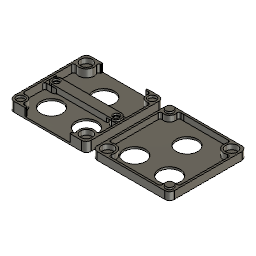
シノン_髪飾り_mk1_v8 (Autodesk Fusion 360 design; units mm, degrees)
Autodesk Fusion 360 part; units mm, degrees
note: some values were not read from the file. Set by a fixed rule: which face or edge a step refers to.
sketch "スケッチ1" plane through (0, 0, 0) normal (0, 0, 1) x (1, 0, 0)
  line L0 (20, 20) -> (-20, 20)
  line L1 (-20, 20) -> (-20, -20)
  line L2 (-20, -20) -> (20, -20)
  line L3 (20, -20) -> (20, 20)
  line L4 (20, 20) -> (-20, -20) construction
  line L5 (-20, 20) -> (20, -20) construction
  circle A0 centre (0, 9) radius 5.5
  circle A1 centre (-9, -9) radius 5.5
  circle A2 centre (9, -9) radius 5.5
  line L6 (0, 0) -> (0, 9) construction
  dimension "d1" = 40
  dimension "d2" = 40
  dimension "d3" = 11
  dimension "d4" = 11
  dimension "d5" = 11
  dimension "d7" = 11
  dimension "d8" = 11
  dimension "d9" = 11
  constraint horizontal L0
  constraint perpendicular L0 L1
  constraint parallel L0 L2
  constraint parallel L1 L3
  constraint coincident L4 L6.start
  constraint coincident L5 L6.start
  constraint coincident L6.start origin
  constraint coincident L4 A1.centre
  constraint coincident L5 A2.centre
  constraint coincident A0.centre L6.end
  constraint vertical L6
  measures "d1" distance of L1.end L2.end
  measures "d2" distance of L0.end L1.end
  measures "d3" diameter of A1
  measures "d4" diameter of A2
  measures "d5" diameter of A0
  measures "d7" distance of L1 A1.centre
  measures "d8" distance of L3 A2.centre
  measures "d9" distance of L0 A0.centre
extrude "押し出し1" add sketch "スケッチ1" along normal blind 4 makes body 1
sketch "スケッチ2" plane through (0, 0, 4) normal (0, 0, 1) x (-1, 0, 0)
  circle A0 centre (0, -9) radius 5.5
  circle A1 centre (9, 9) radius 5.5
  circle A2 centre (-9, 9) radius 5.5
  line L0 (-20, 20) -> (-20, -20)
  line L1 (-20, -20) -> (20, -20)
  line L2 (20, -20) -> (20, 20)
  line L3 (20, 20) -> (-20, 20)
  line L4 (-19, -19) -> (19, -19)
  line L5 (19, -19) -> (19, 19)
  line L6 (19, 19) -> (-19, 19)
  line L7 (-19, 19) -> (-19, -19)
  line L8 (-19, -19) -> (19, 19) construction
  line L9 (19, -19) -> (-19, 19) construction
  dimension "d12" = 1
  dimension "d13" = 1
  constraint horizontal L4
  constraint perpendicular L4 L5
  constraint parallel L4 L6
  constraint parallel L5 L7
  constraint coincident L8 origin
  constraint coincident L9 origin
  measures "d12" distance of L0 L7
  measures "d13" distance of L1 L4
extrude "押し出し2" cut sketch "スケッチ2" against normal blind 3 contours L4 L5 L6 L7 bodies 1
sketch "スケッチ3" plane through (0, 0, 1) normal (0, 0, 1) x (-1, 0, 0)
  circle A0 centre (-9, 9) radius 5.5
  circle A1 centre (0, -9) radius 5.5
  circle A2 centre (9, 9) radius 5.5
  line L0 (-19, 19) -> (-19, -19)
  line L1 (-19, -19) -> (19, -19)
  line L2 (19, -19) -> (19, 19)
  line L3 (19, 19) -> (-19, 19)
  circle A3 centre (15.5, 0) radius 2.5
  line L4 (19, 0) -> (-19, 0) construction
  circle A4 centre (15.5, 0) radius 1.25
  line L5 (20, -20) -> (20, 20)
  line L6 (0, -19) -> (0, 19)
  line L7 (15.5, -2.5) -> (19, -2.5)
  line L8 (15.5, 2.5) -> (19, 2.5)
  circle A5 centre (-15.5, 0) radius 2.5
  circle A6 centre (-15.5, 0) radius 1.25
  line L9 (-15.5, -2.5) -> (-19, -2.5)
  line L10 (-15.5, 2.5) -> (-19, 2.5)
  dimension "d16" = 5
  dimension "d17" = 2.5
  dimension "d19" = 3.5
  constraint midpoint L2 L4.start
  constraint midpoint L0 L4.end
  constraint coincident A3.centre L4
  constraint concentric A3 A4
  constraint midpoint L1 L6.start
  constraint midpoint L3 L6.end
  constraint coincident A3 L7.start
  constraint coincident L2 L7.end
  constraint perpendicular L2 L7
  constraint coincident A3 L8.start
  constraint coincident L2 L8.end
  constraint perpendicular L2 L8
  constraint tangent A3 L7
  constraint tangent A3 L8
  constraint symmetric A3 L6 A5
  constraint symmetric A4 L6 A6
  constraint symmetric L6 L7.start L9.start
  constraint symmetric L6 L7.end L9.end
  constraint symmetric L6 L8.start L10.start
  constraint symmetric L6 L8.end L10.end
  measures "d16" diameter of A3
  measures "d17" diameter of A4
  measures "d19" distance of L2 A3.centre
extrude "押し出し3" add 1 faces at (-6.3333, 19.6667, 4) along direction (0, 0, 1) blind 1 on bodies 1 bodies 1
extrude "押し出し4" add sketch "スケッチ3" along normal blind 3 contours L2 A3 L7 L8 | L0 A5 L9 L10 | A3 | A5 bodies 1
fillet "フィレット1" radius 2 4 edges at (-19, -19, 3) (19, -19, 3) (19, 19, 3) (-19, 19, 3) on bodies 1
fillet "フィレット2" radius 2.5 4 edges at (20, 20, 2.5) (20, -20, 2.5) (-20, 20, 2.5) (-20, -20, 2.5) on bodies 1
sketch "スケッチ5" plane through (0, 0, 5) normal (0, 0, 1) x (-1, 0, 0)
  line L0 (17, -19) -> (-17, -19)
  arc A0 (-19, -17) -> (-17, -19) centre (-17, -17) ccw
  line L1 (-19, -17) -> (-19, 17)
  arc A1 (-17, 19) -> (-19, 17) centre (-17, 17) ccw
  line L2 (-17, 19) -> (17, 19)
  arc A2 (19, 17) -> (17, 19) centre (17, 17) ccw
  line L3 (19, 17) -> (19, -17)
  arc A3 (17, -19) -> (19, -17) centre (17, -17) ccw
  arc A4 (20, 17.5) -> (17.5, 20) centre (17.5, 17.5) ccw
  line L4 (17.5, 20) -> (-17.5, 20)
  arc A5 (-17.5, 20) -> (-20, 17.5) centre (-17.5, 17.5) ccw
  line L5 (-20, 17.5) -> (-20, -17.5)
  arc A6 (-20, -17.5) -> (-17.5, -20) centre (-17.5, -17.5) ccw
  line L6 (-17.5, -20) -> (17.5, -20)
  arc A7 (17.5, -20) -> (20, -17.5) centre (17.5, -17.5) ccw
  line L7 (20, -17.5) -> (20, 17.5)
extrude "押し出し6" cut 2 faces at (-15.867, 0.0689, 1) (15.2939, 0.4998, 1) along direction (0, 0, -1) blind 1 on bodies 1 bodies 1
fillet "フィレット3" radius 1 4 edges at (19, -2.5, 2.5) (19, 2.5, 2.5) (-19, 2.5, 2.5) (-19, -2.5, 2.5) on bodies 1
sketch "スケッチ6" plane through (0, 0, 1) normal (0, 0, 1) x (-1, 0, 0)
  circle A0 centre (0, -9) radius 5.5
  circle A1 centre (9, 9) radius 5.5
  circle A2 centre (-9, 9) radius 5.5
  arc A3 (18, 2.5) -> (19, 3.5) centre (18, 3.5) ccw
  line L0 (19, 3.5) -> (19, 17)
  arc A4 (19, 17) -> (17, 19) centre (17, 17) ccw
  line L1 (17, 19) -> (-17, 19)
  arc A5 (-17, 19) -> (-19, 17) centre (-17, 17) ccw
  line L2 (-19, 17) -> (-19, 3.5)
  arc A6 (-19, 3.5) -> (-18, 2.5) centre (-18, 3.5) ccw
  line L3 (-18, 2.5) -> (-15.5, 2.5)
  arc A7 (-15.5, -2.5) -> (-15.5, 2.5) centre (-15.5, 0) ccw
  line L4 (-15.5, -2.5) -> (-18, -2.5)
  arc A8 (-18, -2.5) -> (-19, -3.5) centre (-18, -3.5) ccw
  line L5 (-19, -3.5) -> (-19, -17)
  arc A9 (-19, -17) -> (-17, -19) centre (-17, -17) ccw
  line L6 (-17, -19) -> (17, -19)
  arc A10 (17, -19) -> (19, -17) centre (17, -17) ccw
  line L7 (19, -17) -> (19, -3.5)
  arc A11 (19, -3.5) -> (18, -2.5) centre (18, -3.5) ccw
  line L8 (18, -2.5) -> (15.5, -2.5)
  arc A12 (15.5, 2.5) -> (15.5, -2.5) centre (15.5, 0) ccw
  line L9 (15.5, 2.5) -> (18, 2.5)
  circle A13 centre (16, -16) radius 3
  circle A14 centre (16, -16) radius 4
  line L10 (0, 0) -> (0, -19)
  line L11 (15.5, 0) -> (-15.5, 0)
  circle A15 centre (-16, 16) radius 3
  circle A16 centre (-16, 16) radius 4
  line L12 (19, 19) -> (-19, 19)
  line L13 (-19, 19) -> (-19, -19)
  line L14 (13.0505, -0.5) -> (-13.0505, -0.5)
  line L15 (13.0505, 0.5) -> (-13.0505, 0.5)
  dimension "d38" = 6
  dimension "d39" = 8
  dimension "d47" = 6
  dimension "d48" = 8
  dimension "d59" = 0.5
  constraint tangent L6 A13
  constraint tangent L7 A13
  constraint concentric A13 A14
  constraint coincident L10.start origin
  constraint midpoint L6 L10.end
  constraint coincident A12.centre L11.start
  constraint coincident A7.centre L11.end
  constraint tangent A15 L12
  constraint tangent A15 L13
  constraint concentric A15 A16
  constraint coincident A12 L14.start
  constraint coincident A7 L14.end
  constraint parallel L11 L14
  constraint symmetric L11 L14.start L15.start
  constraint symmetric L11 L14.end L15.end
  measures "d38" diameter of A13
  measures "d39" diameter of A14
  measures "d47" diameter of A15
  measures "d48" diameter of A16
  measures "d59" distance of L11 L14
extrude "押し出し9" add sketch "スケッチ6" along normal blind 4 contours L6 L7 A13 A14 | L6 A10 L7 A13 | L1 L2 A15 A16 L12 L13 | L1 A5 L2 A15 L12 L13 bodies 1
fillet "フィレット5" radius 1 4 edges at (-19, 13.3542, 3) (-13.3542, 19, 3) (19, -13.3542, 3) (13.3542, -19, 3) on bodies 1
extrude "押し出し10" add sketch "スケッチ6" along normal blind 1.8 contours A13 | A15 bodies 1
sketch "スケッチ7" plane through (0, 0, 5) normal (0, 0, 1) x (-1, 0, 0)
  line L0 (-19, -17) -> (-19, 11.4174)
  line L1 (19, 17) -> (19, -11.4174)
  arc A0 (20, 17.5) -> (17.5, 20) centre (17.5, 17.5) ccw
  line L2 (17.5, 20) -> (-17.5, 20)
  arc A1 (-17.5, 20) -> (-20, 17.5) centre (-17.5, 17.5) ccw
  line L3 (-20, 17.5) -> (-20, -17.5)
  arc A2 (-20, -17.5) -> (-17.5, -20) centre (-17.5, -17.5) ccw
  line L4 (-17.5, -20) -> (17.5, -20)
  arc A3 (17.5, -20) -> (20, -17.5) centre (17.5, -17.5) ccw
  line L5 (20, -17.5) -> (20, 17.5)
  line L6 (11.4174, -20) -> (11.4174, -19)
  line L7 (0, 0) -> (0, -20)
  line L8 (11.4174, -19) -> (-17, -19)
  arc A4 (-19, -17) -> (-17, -19) centre (-17, -17) ccw
  line L9 (-11.4174, 19) -> (17, 19)
  arc A5 (19, 17) -> (17, 19) centre (17, 17) ccw
  arc A6 (17.6, -12.3339) -> (19, -11.4174) centre (18, -11.4174) ccw
  arc A7 (17.6, -12.3339) -> (12.3339, -17.6) centre (16, -16) ccw
  arc A8 (11.4174, -19) -> (12.3339, -17.6) centre (11.4174, -18) ccw
  arc A9 (-17.6, 12.3339) -> (-19, 11.4174) centre (-18, 11.4174) ccw
  arc A10 (-17.6, 12.3339) -> (-12.3339, 17.6) centre (-16, 16) ccw
  arc A11 (-11.4174, 19) -> (-12.3339, 17.6) centre (-11.4174, 18) ccw
  circle A12 centre (-16, 16) radius 3
  circle A13 centre (16, -16) radius 3
  line L10 (-11.4174, -20) -> (-11.4174, -19)
  line L11 (0, 0) -> (-20, 0)
  line L12 (11.4174, 20) -> (11.4174, 19)
  line L13 (-11.4174, 20) -> (-11.4174, 19)
  constraint coincident L4 L6.start
  constraint coincident L7.start L11.start
  constraint midpoint L4 L7.end
  constraint coincident L6.end L8.start
  constraint symmetric L6.start L7 L10.start
  constraint symmetric L6.end L7 L10.end
  constraint midpoint L3 L11.end
  constraint symmetric L6.start L11 L12.start
  constraint symmetric L6.end L11 L12.end
  constraint symmetric L10.start L11 L13.start
  constraint symmetric L10.end L11 L9.start
extrude "押し出し11" cut sketch "スケッチ7" against normal blind 4 contours L4 L7 L8 L10 | L4 L6 L7 L8 | L2 L9 L12 L13 bodies 1
fillet "フィレット6" radius 0.3 8 edges at (-11.4174, -20, 3) (-11.4174, -19, 3) (11.4174, -20, 3) (-11.4174, 19, 3) (11.4174, 19, 3) (11.4174, 20, 3) (-11.4174, 20, 3) (11.4174, -19, 3) on bodies 1
extrude "押し出し12" add sketch "スケッチ6" along normal blind 1 contours A7 L10 L11 L14 | A12 L10 L11 L14 | A7 A12 L11 L15 bodies 1
fillet "フィレット7" radius 1 4 edges at (-13.0505, -0.5, 1.5) (-13.0505, 0.5, 1.5) (13.0505, 0.5, 1.5) (13.0505, -0.5, 1.5) on bodies 1
mirror "ミラー1" about plane through (0, 0, 5) normal (0, 0, 1) of bodies 1 makes body 2
extrude "押し出し13" cut 1 faces at (-17.8603, 0, 6) along direction (0, 0, 1) blind 3 on bodies 2 bodies 2
extrude "押し出し14" cut 1 faces at (17.8603, 0, 6) along direction (0, 0, 1) blind 3 on bodies 2 bodies 2
extrude "押し出し15" cut 1 faces at (4.1126, -0.1667, 8) along direction (0, 0, 1) blind 1 on bodies 2 bodies 2
sketch "スケッチ8" plane through (0, 0, 9) normal (0, 0, -1) x (1, 0, 0)
  line L0 (19, -17) -> (19, 11.4174)
  arc A0 (19, 11.4174) -> (17.6, 12.3339) centre (18, 11.4174) ccw
  arc A1 (12.3339, 17.6) -> (17.6, 12.3339) centre (16, 16) ccw
  arc A2 (12.3339, 17.6) -> (11.6482, 18.973) centre (11.4174, 18) ccw
  arc A3 (11.4174, 19.2649) -> (11.6482, 18.973) centre (11.7174, 19.2649) ccw
  line L1 (11.4174, 19.2649) -> (11.4174, 19.7)
  arc A4 (11.7174, 20) -> (11.4174, 19.7) centre (11.7174, 19.7) ccw
  line L2 (11.7174, 20) -> (-11.7174, 20)
  arc A5 (-11.4174, 19.7) -> (-11.7174, 20) centre (-11.7174, 19.7) ccw
  line L3 (-11.4174, 19.7) -> (-11.4174, 19.3)
  arc A6 (-11.7174, 19) -> (-11.4174, 19.3) centre (-11.7174, 19.3) ccw
  line L4 (-11.7174, 19) -> (-17, 19)
  arc A7 (-17, 19) -> (-19, 17) centre (-17, 17) ccw
  line L5 (-19, 17) -> (-19, -11.4174)
  arc A8 (-19, -11.4174) -> (-17.6, -12.3339) centre (-18, -11.4174) ccw
  arc A9 (-12.3339, -17.6) -> (-17.6, -12.3339) centre (-16, -16) ccw
  arc A10 (-12.3339, -17.6) -> (-11.6482, -18.973) centre (-11.4174, -18) ccw
  arc A11 (-11.4174, -19.2649) -> (-11.6482, -18.973) centre (-11.7174, -19.2649) ccw
  line L6 (-11.4174, -19.2649) -> (-11.4174, -19.7)
  arc A12 (-11.7174, -20) -> (-11.4174, -19.7) centre (-11.7174, -19.7) ccw
  line L7 (-11.7174, -20) -> (11.7174, -20)
  arc A13 (11.4174, -19.7) -> (11.7174, -20) centre (11.7174, -19.7) ccw
  line L8 (11.4174, -19.7) -> (11.4174, -19.3)
  arc A14 (11.7174, -19) -> (11.4174, -19.3) centre (11.7174, -19.3) ccw
  line L9 (11.7174, -19) -> (17, -19)
  arc A15 (17, -19) -> (19, -17) centre (17, -17) ccw
  circle A16 centre (15.5, 0) radius 1.25
  circle A17 centre (0, -9) radius 5.5
  circle A18 centre (-15.5, 0) radius 1.25
  circle A19 centre (-9, 9) radius 5.5
  circle A20 centre (9, 9) radius 5.5
  circle A21 centre (-15.5, 0) radius 1.25
  circle A22 centre (15.5, 0) radius 1.25
  line L10 (-11.7174, 19) -> (11.6482, 18.973)
  line L11 (-11.6482, -18.973) -> (11.7174, -19)
  constraint concentric A18 A21
  constraint concentric A16 A22
  constraint coincident A6.start L4.start
  constraint coincident A2.end A3.end
  constraint coincident A10.end A11.end
  constraint coincident A14.start L9.start
extrude "押し出し16" add sketch "スケッチ8" along normal blind 4 contours A11 L6 A12 L7 A13 L8 A14 L11 | A3 L1 A4 L2 A5 L3 A6 L10 bodies 2
fillet "フィレット8" radius 1 1 edges at (11.6482, -18.973, 7) on bodies 2
fillet "フィレット9" radius 1 1 edges at (-11.6482, 18.973, 7) on bodies 2
extrude "押し出し17" add sketch "スケッチ8" against normal blind 1 contours A16 A22 | A18 A21 bodies 2
extrude "押し出し18" cut 1 faces at (3.8023, -19.6578, 5) along direction (0, 0, 1) blind 1 on bodies 2 bodies 2
sketch "スケッチ9" plane through (0, 0, 9) normal (0, 0, -1) x (1, 0, 0)
  arc A0 (-12.3247, -17.5786) -> (-11.407, -18.9733) centre (-11.4059, -17.9733) ccw
  line L0 (-11.407, -18.9733) -> (11.7174, -19)
  line L1 (11.7174, -19) -> (17, -19)
  arc A1 (17, -19) -> (19, -17) centre (17, -17) ccw
  line L2 (19, -17) -> (19, 11.4174)
  arc A2 (19, 11.4174) -> (17.6, 12.3339) centre (18, 11.4174) ccw
  arc A3 (12.3247, 17.5786) -> (17.6, 12.3339) centre (16, 16) ccw
  arc A4 (12.3247, 17.5786) -> (11.407, 18.9733) centre (11.4059, 17.9733) ccw
  line L3 (11.407, 18.9733) -> (-11.7174, 19)
  line L4 (-11.7174, 19) -> (-17, 19)
  arc A5 (-17, 19) -> (-19, 17) centre (-17, 17) ccw
  line L5 (-19, 17) -> (-19, -11.4174)
  arc A6 (-19, -11.4174) -> (-17.6, -12.3339) centre (-18, -11.4174) ccw
  arc A7 (-12.3247, -17.5786) -> (-17.6, -12.3339) centre (-16, -16) ccw
  circle A8 centre (0, -9) radius 5.5
  circle A9 centre (-9, 9) radius 5.5
  circle A10 centre (9, 9) radius 5.5
  line L6 (-19, -5) -> (-17.9, -5)
  line L7 (-17.9, -5) -> (-17.9, 20)
  line L8 (-11.7174, 19) -> (-11.7174, 17.9)
  line L9 (-11.7174, 17.9) -> (-17.9, 17.9)
  line L10 (-12.7174, 17.9) -> (-12.7174, 19)
  dimension "d82" = 1.1
  dimension "d83" = 1.1
  dimension "d88" = 1
  constraint coincident L5 L6.start
  constraint perpendicular L5 L6
  constraint perpendicular L6 L7
  constraint coincident L3.end L4.start
  constraint perpendicular L4 L8
  constraint coincident L7 L9.end
  constraint perpendicular L7 L9
  constraint coincident L9 L10.start
  constraint coincident L4 L10.end
  constraint perpendicular L4 L10
  measures "d82" distance of L6.start L6.end
  measures "d83" distance of L3.end L8.end
  measures "d88" distance of L8 L10
extrude "押し出し19" add sketch "スケッチ9" along normal blind 4 separate body contours A5 L5 L6 L7 | L4 A5 L7 L9 L10 makes body 3
fillet "フィレット10" radius 1 1 edges at (-17.9, -17.9, 7) on bodies 3
pattern_circular "C パターン1" count 2 over 360 about axis through (0, 0, 1.75) along (0, 0, 1) of bodies 3 makes body 4
combine "結合1" operation add target body 3 tool bodies 4 2
extrude "押し出し20" cut 2 faces at (-16.293, 15.3862, 2.8) (15.2714, -14.5885, 2.8) along direction (0, 0, -1) blind 0.4 on bodies 1 bodies 1
extrude "押し出し21" cut 2 faces at (15.2714, -14.5885, 7.2) (-16.293, 15.3862, 7.2) along direction (0, 0, 1) blind 1.4 on bodies 3 bodies 3
extrude "押し出し24" cut 2 faces at (-18.6333, -9.6333, 5) (18.6333, 9.6333, 5) along direction (0, 0, 1) blind 4 on bodies 3 bodies 3
sketch "スケッチ10" plane through (0, 0, 1) normal (0, 0, 1) x (-1, 0, 0)
  arc A0 (-12.3377, -0.5) -> (-13.2412, -1.0714) centre (-12.3377, -1.5) ccw
  arc A1 (-15.5, -2.5) -> (-13.2412, -1.0714) centre (-15.5, 0) ccw
  line L0 (-15.5, -2.5) -> (-18, -2.5)
  arc A2 (-18, -2.5) -> (-19, -3.5) centre (-18, -3.5) ccw
  line L1 (-19, -3.5) -> (-19, -17)
  arc A3 (-19, -17) -> (-17, -19) centre (-17, -17) ccw
  line L2 (-17, -19) -> (-11.7174, -19)
  arc A4 (-11.4174, -19.3) -> (-11.7174, -19) centre (-11.7174, -19.3) ccw
  line L3 (-11.4174, -19.3) -> (-11.4174, -19.7)
  arc A5 (-11.7174, -20) -> (-11.4174, -19.7) centre (-11.7174, -19.7) ccw
  line L4 (-11.7174, -20) -> (11.7174, -20)
  arc A6 (11.4174, -19.7) -> (11.7174, -20) centre (11.7174, -19.7) ccw
  line L5 (11.4174, -19.7) -> (11.4174, -19.2649)
  arc A7 (11.6482, -18.973) -> (11.4174, -19.2649) centre (11.7174, -19.2649) ccw
  arc A8 (11.6482, -18.973) -> (12.3339, -17.6) centre (11.4174, -18) ccw
  arc A9 (17.6, -12.3339) -> (12.3339, -17.6) centre (16, -16) ccw
  arc A10 (17.6, -12.3339) -> (19, -11.4174) centre (18, -11.4174) ccw
  line L6 (19, -11.4174) -> (19, -3.5)
  arc A11 (19, -3.5) -> (18, -2.5) centre (18, -3.5) ccw
  line L7 (18, -2.5) -> (15.5, -2.5)
  arc A12 (13.2412, -1.0714) -> (15.5, -2.5) centre (15.5, 0) ccw
  arc A13 (13.2412, -1.0714) -> (12.3377, -0.5) centre (12.3377, -1.5) ccw
  line L8 (12.3377, -0.5) -> (-12.3377, -0.5)
  circle A14 centre (0, -9) radius 5.5
  circle A15 centre (-17, -17) radius 2
  circle A16 centre (-17, -17) radius 3
  line L9 (-20, 17.5) -> (-20, -17.5)
  line L10 (-17.5, -20) -> (-11.7174, -20)
  dimension "d104" = 4
  dimension "d105" = 6
  dimension "d106" = 3
  dimension "d107" = 3
  constraint concentric A15 A16
  measures "d104" diameter of A15
  measures "d105" diameter of A16
  measures "d106" distance of A3.centre L9
  measures "d107" distance of A3.centre L10
extrude "押し出し25" add sketch "スケッチ10" along normal blind 4 contours L1 L2 A15 A16 bodies 1
extrude "押し出し26" add 1 faces at (17.5842, 16.9811, 1) along direction (0, 0, 1) blind 2.8 on bodies 1 bodies 1
fillet "フィレット12" radius 1 2 edges at (14.7639, 19, 3) (19, 14.7639, 3) on bodies 1
sketch "スケッチ11" plane through (0, 0, 1) normal (0, 0, 1) x (-1, 0, 0)
  arc A0 (-13.2412, 1.0714) -> (-12.3377, 0.5) centre (-12.3377, 1.5) ccw
  line L0 (-12.3377, 0.5) -> (12.3377, 0.5)
  arc A1 (12.3377, 0.5) -> (13.2412, 1.0714) centre (12.3377, 1.5) ccw
  arc A2 (15.5, 2.5) -> (13.2412, 1.0714) centre (15.5, 0) ccw
  line L1 (15.5, 2.5) -> (18, 2.5)
  arc A3 (18, 2.5) -> (19, 3.5) centre (18, 3.5) ccw
  line L2 (19, 3.5) -> (19, 17)
  arc A4 (19, 17) -> (17, 19) centre (17, 17) ccw
  line L3 (17, 19) -> (11.7174, 19)
  arc A5 (11.4174, 19.3) -> (11.7174, 19) centre (11.7174, 19.3) ccw
  line L4 (11.4174, 19.3) -> (11.4174, 19.7)
  arc A6 (11.7174, 20) -> (11.4174, 19.7) centre (11.7174, 19.7) ccw
  line L5 (11.7174, 20) -> (-11.7174, 20)
  arc A7 (-11.4174, 19.7) -> (-11.7174, 20) centre (-11.7174, 19.7) ccw
  line L6 (-11.4174, 19.7) -> (-11.4174, 19.2649)
  arc A8 (-11.6482, 18.973) -> (-11.4174, 19.2649) centre (-11.7174, 19.2649) ccw
  arc A9 (-11.6482, 18.973) -> (-12.3339, 17.6) centre (-11.4174, 18) ccw
  arc A10 (-17.6, 12.3339) -> (-12.3339, 17.6) centre (-16, 16) ccw
  arc A11 (-17.6, 12.3339) -> (-19, 11.4174) centre (-18, 11.4174) ccw
  line L7 (-19, 11.4174) -> (-19, 3.5)
  arc A12 (-19, 3.5) -> (-18, 2.5) centre (-18, 3.5) ccw
  line L8 (-18, 2.5) -> (-15.5, 2.5)
  arc A13 (-13.2412, 1.0714) -> (-15.5, 2.5) centre (-15.5, 0) ccw
  circle A14 centre (9, 9) radius 5.5
  circle A15 centre (-9, 9) radius 5.5
  circle A16 centre (17, 17) radius 2
  circle A17 centre (17, 17) radius 3
  line L9 (20, -17.5) -> (20, 17.5)
  line L10 (17.5, 20) -> (11.7174, 20)
  dimension "d114" = 4
  dimension "d115" = 6
  dimension "d116" = 3
  dimension "d117" = 3
  constraint concentric A16 A17
  measures "d114" diameter of A16
  measures "d115" diameter of A17
  measures "d116" distance of A4.centre L9
  measures "d117" distance of A4.centre L10
extrude "押し出し27" add sketch "スケッチ11" along normal blind 4 contours L2 L3 A16 A17 bodies 1
extrude "押し出し28" add 1 faces at (-16.6888, -17.8732, 1) along direction (0, 0, 1) blind 2.8 on bodies 1 bodies 1
fillet "フィレット13" radius 1 2 edges at (-14.7639, -19, 3) (-19, -14.7639, 3) on bodies 1
sketch "スケッチ12" plane through (0, 0, 9) normal (0, 0, -1) x (1, 0, 0)
  line L0 (-19, 17) -> (-19, -11.4174)
  arc A0 (-19, -11.4174) -> (-17.6, -12.3339) centre (-18, -11.4174) ccw
  arc A1 (-12.3247, -17.5786) -> (-17.6, -12.3339) centre (-16, -16) ccw
  arc A2 (-12.3247, -17.5786) -> (-11.407, -18.9733) centre (-11.4059, -17.9733) ccw
  line L1 (-11.407, -18.9733) -> (11.7174, -19)
  line L2 (11.7174, -19) -> (17, -19)
  arc A3 (17, -19) -> (19, -17) centre (17, -17) ccw
  line L3 (19, -17) -> (19, 11.4174)
  arc A4 (19, 11.4174) -> (17.6, 12.3339) centre (18, 11.4174) ccw
  arc A5 (12.3247, 17.5786) -> (17.6, 12.3339) centre (16, 16) ccw
  arc A6 (12.3247, 17.5786) -> (11.407, 18.9733) centre (11.4059, 17.9733) ccw
  line L4 (11.407, 18.9733) -> (-11.7174, 19)
  line L5 (-11.7174, 19) -> (-17, 19)
  arc A7 (-17, 19) -> (-19, 17) centre (-17, 17) ccw
  circle A8 centre (9, 9) radius 5.5
  circle A9 centre (-9, 9) radius 5.5
  circle A10 centre (0, -9) radius 5.5
  circle A11 centre (17, -17) radius 2
  line L6 (20, 17.5) -> (20, -17.5)
  line L7 (17.5, -20) -> (-17.5, -20)
  circle A12 centre (-17, 17) radius 2
  line L8 (-17.5, 20) -> (17.5, 20)
  line L9 (-20, -17.5) -> (-20, 17.5)
  circle A13 centre (-17, 17) radius 3
  circle A14 centre (17, -17) radius 3
  dimension "d124" = 4
  dimension "d125" = 3
  dimension "d126" = 3
  dimension "d127" = 4
  dimension "d128" = 3
  dimension "d130" = 3
  dimension "d138" = 6
  dimension "d139" = 6
  constraint concentric A12 A13
  constraint concentric A11 A14
  measures "d124" diameter of A11
  measures "d125" distance of A3.centre L6
  measures "d126" distance of A3.centre L7
  measures "d127" diameter of A12
  measures "d128" distance of A7.centre L8
  measures "d130" distance of A7.centre L9
  measures "d138" diameter of A13
  measures "d139" diameter of A14
extrude "押し出し29" add sketch "スケッチ12" along normal blind 4 contours A7 A12 | A3 A11 bodies 3
extrude "押し出し30" add sketch "スケッチ12" along normal blind 3 contours L0 L5 A12 A13 | L2 L3 A11 A14 bodies 3
fillet "フィレット16" radius 1 4 edges at (-19, -14.7639, 7.5) (-14.7639, -19, 7.5) (19, 14.7639, 7.5) (14.7639, 19, 7.5) on bodies 3
move_body "移動3" bodies 3 to x (1, 0, 0) y (0, -1, 0) z (0, 0, -1) at (0, -43, 10)
move_face "面をオフセット2" offset -0.05 4 faces at (-18.9975, -17.0997, 4.2) (15.0023, 17.0952, 4.6) (18.5721, 18.2363, 4.6) (16.1774, 15.177, 4.6) on bodies 1
move_body "移動4" bodies 3 to x (-1, 0, 0) y (0, -1, 0) z (0, 0, 1) at (43, -43, 0)
sketch "スケッチ13" plane through (0, 0, 4) normal (0, 0, 1) x (-1, 0, 0)
  circle A0 centre (15.5, 0) radius 1.25
  line L0 (15.5, -2.5) -> (18, -2.5)
  arc A1 (19, -3.5) -> (18, -2.5) centre (18, -3.5) ccw
  line L1 (19, -3.5) -> (19, 3.5)
  arc A2 (18, 2.5) -> (19, 3.5) centre (18, 3.5) ccw
  line L2 (18, 2.5) -> (15.5, 2.5)
  arc A3 (15.5, 2.5) -> (15.5, -2.5) centre (15.5, 0) ccw
  line L3 (17.5, 20) -> (-17.5, 20)
  arc A4 (20, 17.5) -> (17.5, 20) centre (17.5, 17.5) ccw
  line L4 (20, -17.5) -> (20, 17.5)
  arc A5 (17.5, -20) -> (20, -17.5) centre (17.5, -17.5) ccw
  line L5 (-17.5, -20) -> (17.5, -20)
  arc A6 (-17.5, 20) -> (-20, 17.5) centre (-17.5, 17.5) ccw
  line L6 (-20, 17.5) -> (-20, -17.5)
  arc A7 (-20, -17.5) -> (-17.5, -20) centre (-17.5, -17.5) ccw
  circle A8 centre (-15.5, 0) radius 1.25
  circle A9 centre (15.5, 0) radius 1.25
  circle A10 centre (9, 9) radius 5.5
  circle A11 centre (-9, 9) radius 5.5
  circle A12 centre (0, -9) radius 5.5
  circle A13 centre (15.5, 0) radius 1.65
  circle A14 centre (-15.5, 0) radius 1.65
  circle A15 centre (15.5, 0) radius 2.5
  circle A16 centre (-15.5, 0) radius 2.5
  line L7 (15.5, -2.5) -> (-15.5, -2.5)
  line L8 (15.5, 2.5) -> (-15.5, 2.5)
  line L9 (13.2087, -1) -> (-13.2087, -1)
  line L10 (13.2087, 1) -> (-13.2087, 1)
  circle A17 centre (15.5, 0) radius 2.75
  circle A18 centre (-15.5, 0) radius 2.75
  dimension "d144" = 3.3
  dimension "d145" = 3.3
  dimension "d146" = 5
  dimension "d147" = 5
  dimension "d148" = 1.5
  dimension "d149" = 1.5
  dimension "d150" = 5.5
  dimension "d151" = 5.5
  constraint concentric A9 A13
  constraint concentric A8 A14
  constraint concentric A13 A15
  constraint concentric A14 A16
  constraint horizontal L7
  constraint coincident A15 L0.start
  constraint coincident A16 L7.end
  constraint horizontal L8
  constraint tangent A15 L8
  constraint coincident A15 L2.end
  constraint coincident A16 L8.end
  constraint tangent A16 L7
  constraint coincident A15 L9.start
  constraint coincident A16 L9.end
  constraint horizontal L9
  constraint coincident A15 L10.start
  constraint coincident A16 L10.end
  constraint parallel L8 L10
  constraint concentric A15 A17
  constraint concentric A16 A18
  measures "d144" diameter of A13
  measures "d145" diameter of A14
  measures "d146" diameter of A15
  measures "d147" diameter of A16
  measures "d148" distance of L7 L9
  measures "d149" distance of L8 L10
  measures "d150" diameter of A17
  measures "d151" diameter of A18
extrude "押し出し31" add sketch "スケッチ13" along normal blind 1 separate body contours A3 A15 L7 L9 A17 | A3 A15 | A3 A15 L9 L10 A17 | L7 L9 A17 A18 | A3 A15 L8 L10 A17 | L9 L10 A17 A18 | A16 L7 L9 A18 | L8 L10 A17 A18 | A16 L9 L10 A18 | A16 | A16 L8 L10 A18 makes body 5
extrude "押し出し32" add sketch "スケッチ13" against normal blind 2 contours L7 L9 A17 A18 | L8 L10 A17 A18 bodies 5
fillet "フィレット17" radius 0.5 8 edges at (-14.3544, -2.5, 3) (-14.3544, 2.5, 3) (-12.9383, 1, 3) (14.3544, -2.5, 3) (14.3544, 2.5, 3) (12.9383, 1, 3) (-12.9383, -1, 3) (12.9383, -1, 3) on bodies 5
equation "d3 = d4"
equation "d5 = d4"
equation "d9 = d8"
equation "d146 = d147"
